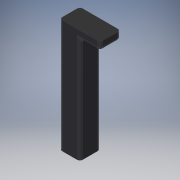
# Autodesk Inventor part: TableLeg
Saved by Autodesk Inventor 2018 (Build 220112000, 112)
## iProperties
Created: 2018-02-18
Part Number: TableLeg
Material: Generic
Document SubType Name: Modeling
Designer: reide
Density: 1 g/cm^3
Appearance: Default
Author: reide
Autodesk Inventor part; units mm, degrees
ref_plane "YZ Plane" through (0, 0, 0) normal (1, 0, 0) x (0, 1, 0)
ref_plane "XZ Plane" through (0, 0, 0) normal (0, 1, 0) x (-1, 0, 0)
sketch "Sketch1" plane through (0, 0, 0) normal (0, 0, 1) x (1, 0, 0)
  line L0 (79.395, -155.8766) -> (79.395, 6.5) projected
  line L1 (-8.605, 6.5) -> (-8.605, -107.0766) projected
  line L2 (69.9453, -18.7158) -> (55.4353, -18.7158) projected
  line L3 (79.395, -18.7158) -> (79.395, -23.7158)
  line L4 (79.395, -23.7158) -> (71.895, -23.7158)
  line L5 (71.895, -23.7158) -> (71.895, -31.2158)
  line L6 (71.895, -31.2158) -> (79.395, -31.2158)
  line L7 (79.395, -31.2158) -> (79.395, -23.7158)
  point P0 (0, 0)
  dimension "d0" = 5
  dimension "d1" = 7.5
  dimension "d2" = 7.5
  constraints: 10 end point, 2 parallel, 2 point on line, 1 horizontal, 1 perpendicular
  measures "d0" distance of L3.start L3.end
  measures "d1" distance of L3.end L4.end
  measures "d2" distance of L4.end L5.end
ref_plane "Work Plane1" through (-121.6053, -233.9347, 42.0294) normal (0, 0, -1) x (0, 1, 0)
extrude "Extrusion1" add sketch "Sketch1" along normal up to surface (42.0294 mm away)
sketch "Sketch2" plane through (71.895, -23.7158, 42.0294) normal (0, 0, 1) x (1, 0, 0)
  line L0 (7.5, 0) -> (0, 0) projected
  line L1 (0, 0) -> (15, 0)
  line L2 (15, 0) -> (15, -7.5)
  line L3 (15, -7.5) -> (0, -7.5)
  line L4 (0, -7.5) -> (0, 0)
  point P0 (-71.895, 23.7158)
  dimension "d5" = 15
  constraints: 8 end point, 2 parallel, 1 horizontal, 1 perpendicular
  measures "d5" distance of L2.end L3.end
extrude "Extrusion2" add sketch "Sketch2" against normal blind 3
fillet "Fillet1" radius 1 6 edges at (79.395, -23.7158, 19.5147) (71.895, -23.7158, 21.0147) (79.395, -31.2158, 19.5147) (71.895, -31.2158, 21.0147) (86.895, -23.7158, 40.5294) (86.895, -31.2158, 40.5294)
fillet "Fillet2" radius 1 5 edges at (86.6021, -30.9229, 39.0294) (78.895, -31.2158, 39.0294) (86.6021, -24.0087, 39.0294) (78.895, -23.7158, 39.0294) (86.895, -27.4658, 39.0294)
fillet "Fillet3" radius 1 1 edges at (79.395, -27.4658, 39.0294)
body "Solid1"
